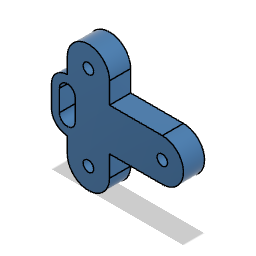
3d10 v1 (Autodesk Fusion 360 design; units mm, degrees)
Autodesk Fusion 360 part; units mm, degrees
sketch "Sketch1" plane through (0, 0, 0) normal (0, 0, 1) x (1, 0, 0)
  circle A0 centre (0, 80) radius 10
  circle A1 centre (0, 80) radius 15
  circle A2 centre (70, 40) radius 10
  circle A3 centre (70, 40) radius 15
  circle A4 centre (0, 0) radius 10
  circle A5 centre (0, 0) radius 15
  line L0 (20, 60) -> (70, 60)
  arc A6 (20, 80) -> (-20, 80) centre (0, 80) ccw
  arc A7 (-20, 0) -> (20, 0) centre (0, 0) ccw
  line L1 (20, 20) -> (70, 20)
  arc A8 (70, 20) -> (70, 60) centre (70, 40) ccw
  line L2 (20, 80) -> (20, 60)
  line L3 (20, 20) -> (20, 0)
  line L4 (-35, 50) -> (-35, 30)
  arc A9 (-35, 30) -> (-20, 15) centre (-20, 30) ccw
  arc A10 (-20, 65) -> (-35, 50) centre (-20, 50) ccw
  line L5 (-20, 80) -> (-20, 65)
  line L6 (-20, 15) -> (-20, 0)
  line L7 (-12.5, 50) -> (-12.5, 30)
  line L8 (-27.5, 50) -> (-27.5, 30)
  arc A11 (-12.5, 50) -> (-27.5, 50) centre (-20, 50) ccw
  arc A12 (-27.5, 30) -> (-12.5, 30) centre (-20, 30) ccw
  dimension "d1" = 20
  dimension "d2" = 30
  dimension "d3" = 40
  dimension "d4" = 20
  dimension "d5" = 30
  dimension "d6" = 40
  dimension "d7" = 20
  dimension "d8" = 30
  dimension "d9" = 40
  dimension "d10" = 80
  dimension "d11" = 40
  dimension "d12" = 70
  dimension "d13" = 40
  dimension "d14" = 20
  dimension "d16" = 30
  dimension "d18" = 30
  dimension "d19" = 20
  dimension "d20" = 20
  dimension "d21" = 30
  dimension "d22" = 15
  dimension "d23" = 15
  dimension "d24" = 20
  dimension "d25" = 30
  dimension "d27" = 12.5
  dimension "d28" = 27.5
  constraint concentric A0 A1
  constraint concentric A0 A6
  constraint concentric A2 A3
  constraint concentric A3 A8
  constraint concentric A4 A5
  constraint concentric A4 A7
  constraint vertical A4.centre A0.centre
  constraint vertical A0.centre A4.centre
  constraint coincident A4.centre A5.centre
  constraint vertical L2
  constraint parallel L2 L5
  constraint tangent L0 A8
  constraint tangent A7 L2
  constraint tangent A6 L5
  constraint coincident L1.start L2
  constraint collinear L2 L3
  constraint vertical L4
  constraint tangent L4 A10
  constraint collinear L5 L6
  constraint vertical A10.centre A9.centre
  constraint coincident A10.centre A11.centre
  constraint vertical L7
  constraint tangent L7 A11
  measures "d1" diameter of A0
  measures "d2" diameter of A1
  measures "d3" diameter of A6
  measures "d4" diameter of A2
  measures "d5" diameter of A3
  measures "d6" diameter of A8
  measures "d7" diameter of A4
  measures "d8" diameter of A5
  measures "d9" diameter of A7
  measures "d10" distance of A0.centre A4.centre
  measures "d11" vertical distance of A2.centre A4.centre
  measures "d12" horizontal distance of A2.centre A4.centre
  measures "d13" distance of L0 L1
  measures "d14" distance of A4.centre L1
  measures "d16" diameter of A10
  measures "d18" diameter of A9
  measures "d19" vertical distance of A10.centre A9.centre
  measures "d20" horizontal distance of A4.centre A9.centre
  measures "d21" vertical distance of A4.centre A9.centre
  measures "d22" diameter of A11
  measures "d23" diameter of A12
  measures "d24" vertical distance of A10.centre A9.centre
  measures "d25" vertical distance of A4.centre A9.centre
  measures "d27" distance of A4.centre L7
  measures "d28" distance of A4.centre L8
extrude "Extrude1" add sketch "Sketch1" along normal mid plane 20 contours A1 | A3 | A5 | L0 A6 A7 L1 A8 L2 L3 L4 A9 A10 L5 L6
sketch "Sketch2" plane through (0, 0, 10) normal (0, 0, 1) x (1, 0, 0)
  circle A0 centre (0, 0) radius 10
  circle A1 centre (0, 80) radius 10
  circle A2 centre (70, 40) radius 10
  arc A3 (-12.5, 50) -> (-27.5, 50) centre (-20, 50) ccw
  line L0 (-12.5, 50) -> (-12.5, 30)
  arc A4 (-27.5, 30) -> (-12.5, 30) centre (-20, 30) ccw
  line L1 (-27.5, 30) -> (-27.5, 50)
  arc A5 (20, 80) -> (-20, 80) centre (0, 80) ccw
  line L2 (-20, 80) -> (-20, 65)
  arc A6 (-20, 65) -> (-35, 50) centre (-20, 50) ccw
  line L3 (-35, 50) -> (-35, 30)
  arc A7 (-35, 30) -> (-20, 15) centre (-20, 30) ccw
  line L4 (-20, 15) -> (-20, 0)
  arc A8 (-20, 0) -> (20, 0) centre (0, 0) ccw
  line L5 (20, 0) -> (20, 20)
  line L6 (20, 20) -> (70, 20)
  arc A9 (70, 20) -> (70, 60) centre (70, 40) ccw
  line L7 (70, 60) -> (20, 60)
  line L8 (20, 60) -> (20, 80)
  circle A10 centre (0, 80) radius 5
  circle A11 centre (70, 40) radius 5
  circle A12 centre (0, 0) radius 5
  dimension "d31" = 10
  dimension "d32" = 10
  dimension "d33" = 10
  constraint concentric A1 A10
  constraint concentric A2 A11
  constraint concentric A0 A12
  measures "d31" diameter of A10
  measures "d32" diameter of A11
  measures "d33" diameter of A12
extrude "Extrude2" add sketch "Sketch2" against normal blind 10 contours A0 | A1 | A2
